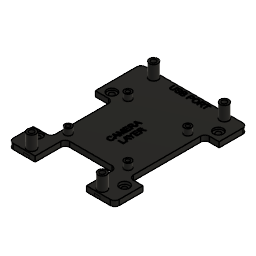
BATTERY-CAMERA_SPACER (Autodesk Fusion 360 design; units mm, degrees)
part number: 2026-05-13-14-17-40-466
Autodesk Fusion 360 part; units mm, degrees
note: some values were not read from the file. Chosen so that the rebuilt part matches the saved one: that a step has no effect; the layout of a text.
sketch "Sketch1" plane through (0, 0, 0) normal (0, 0, 1) x (1, 0, 0)
  line L0 (2.5, 0) -> (57.5, 0)
  line L1 (60, 2.5) -> (60, 72.5)
  line L2 (57.5, 75) -> (2.5, 75)
  line L3 (0, 72.5) -> (0, 2.5)
  arc A0 (2.5, 75) -> (0, 72.5) centre (2.5, 72.5) ccw
  arc A1 (60, 72.5) -> (57.5, 75) centre (57.5, 72.5) ccw
  arc A2 (57.5, 0) -> (60, 2.5) centre (57.5, 2.5) ccw
  arc A3 (0, 2.5) -> (2.5, 0) centre (2.5, 2.5) ccw
  point P0 (60, 0)
  point P1 (0, 75)
  dimension "d1" = 60
  dimension "d2" = 75
  dimension "d3" = 2.5
  constraint horizontal L0
  constraint vertical L1
  constraint horizontal L2
  constraint vertical L3
  constraint coincident P1 L2
  constraint coincident P1 L3
  constraint tangent L2 A0
  constraint tangent L3 A0
  constraint tangent L1 A1
  constraint tangent L2 A1
  constraint equal A0 A1
  constraint coincident P0 L0
  constraint coincident P0 L1
  constraint tangent L0 A2
  constraint tangent L1 A2
  constraint equal A0 A2
  constraint coincident origin L0
  constraint coincident origin L3
  constraint tangent L0 A3
  constraint tangent L3 A3
  constraint equal A0 A3
  measures "d1" distance of origin P0
  measures "d2" distance of origin P1
  measures "d3" radius of A0
extrude "Extrude1" add sketch "Sketch1" along normal blind 3
sketch "Sketch2" plane through (0, 0, 3) normal (0, 0, 1) x (-1, 0, 0)
  arc A0 (0, -2.5) -> (-2.5, 0) centre (-2.5, -2.5) ccw
  line L0 (-2.5, 0) -> (-57.5, 0)
  arc A1 (-57.5, 0) -> (-60, -2.5) centre (-57.5, -2.5) ccw
  line L1 (-60, -2.5) -> (-60, -72.5)
  arc A2 (-60, -72.5) -> (-57.5, -75) centre (-57.5, -72.5) ccw
  line L2 (-57.5, -75) -> (-2.5, -75)
  arc A3 (-2.5, -75) -> (0, -72.5) centre (-2.5, -72.5) ccw
  line L3 (0, -72.5) -> (0, -2.5)
  circle A4 centre (-50, -72) radius 1.4
  circle A5 centre (-50, -72) radius 2.5
  circle A6 centre (-10, -72) radius 1.4
  circle A7 centre (-10, -72) radius 2.5
  circle A8 centre (-50, -3) radius 1.4
  circle A9 centre (-50, -3) radius 2.5
  circle A10 centre (-10, -3) radius 1.4
  circle A11 centre (-10, -3) radius 2.5
  dimension "d6" = 2.8
  dimension "d7" = 5
  dimension "d8" = 10
  dimension "d9" = 3
  dimension "d10" = 2.8
  dimension "d11" = 5
  dimension "d12" = 3
  dimension "d13" = 10
  dimension "d14" = 2.8
  dimension "d15" = 5
  dimension "d16" = 3
  dimension "d17" = 10
  dimension "d18" = 2.8
  dimension "d19" = 5
  dimension "d20" = 10
  dimension "d21" = 3
  constraint concentric A4 A5
  constraint concentric A6 A7
  constraint concentric A8 A9
  constraint concentric A10 A11
  measures "d6" diameter of A4
  measures "d7" diameter of A5
  measures "d8" distance of L1 A4.centre
  measures "d9" distance of L2 A4.centre
  measures "d10" diameter of A6
  measures "d11" diameter of A7
  measures "d12" distance of L2 A6.centre
  measures "d13" distance of L3 A6.centre
  measures "d14" diameter of A8
  measures "d15" diameter of A9
  measures "d16" distance of L0 A8.centre
  measures "d17" distance of L1 A8.centre
  measures "d18" diameter of A10
  measures "d19" diameter of A11
  measures "d20" distance of L3 A10.centre
  measures "d21" distance of L0 A10.centre
extrude "Extrude2" cut sketch "Sketch2" against normal blind 6 contours A4 | A6 | A8 | A10
extrude "Extrude3" add sketch "Sketch2" along normal blind 8 contours A5 | A7 | A9 | A11
sketch "Sketch3" plane through (0, 0, 3) normal (0, 0, 1) x (-1, 0, 0)
  line L0 (-17, -70) -> (-44, -70) construction
  line L1 (-44, -70) -> (-44, -75) construction
  line L2 (-44, -75) -> (-17, -75) construction
  line L3 (-17, -75) -> (-17, -70) construction
  line L4 (-36.7995, -28.0303) -> (-36.8426, -50.0364) construction
  line L5 (-36.8426, -50.0364) -> (-24.5082, -50.0606) construction
  line L6 (-24.5082, -50.0606) -> (-24.4651, -28.0545) construction
  line L7 (-24.4651, -28.0545) -> (-36.7995, -28.0303) construction
  dimension "d26" = 3
  dimension "d28" = 3
  text T0 "USB PORT" font "Arial" height 3 align centre middle in box 27 x 5 at (-17, -70) x (-1, 0) y (0, -1) spacing 1
extrude "Extrude4" [no effect]
sketch "Sketch13" plane through (0, 0, 3) normal (0, 0, 1) x (-1, 0, 0)
  circle A0 centre (-5.4, -11) radius 1.4
  circle A1 centre (-5.4, -11) radius 2.75
  line L0 (0, -72.5) -> (0, -2.5)
  line L1 (-2.5, 0) -> (-57.5, 0)
  circle A2 centre (-54.6, -11) radius 1.4
  circle A3 centre (-54.6, -11) radius 2.75
  line L2 (-60, -2.5) -> (-60, -72.5)
  circle A4 centre (-5.4, -53) radius 1.4
  circle A5 centre (-5.4, -53) radius 2.75
  line L3 (-57.5, -75) -> (-2.5, -75)
  circle A6 centre (-54.6, -64) radius 1.4
  circle A7 centre (-54.6, -64) radius 2.75
  dimension "d67" = 2.8
  dimension "d68" = 5.5
  dimension "d69" = 5.4
  dimension "d70" = 11
  dimension "d71" = 2.8
  dimension "d72" = 5.5
  dimension "d73" = 11
  dimension "d74" = 5.4
  dimension "d75" = 2.8
  dimension "d76" = 5.5
  dimension "d77" = 5.4
  dimension "d78" = 22
  dimension "d79" = 2.8
  dimension "d80" = 5.5
  dimension "d81" = 5.4
  dimension "d82" = 11
  constraint concentric A0 A1
  constraint concentric A2 A3
  constraint concentric A4 A5
  constraint concentric A6 A7
  measures "d67" diameter of A0
  measures "d68" diameter of A1
  measures "d69" distance of A0.centre L0
  measures "d70" distance of A0.centre L1
  measures "d71" diameter of A2
  measures "d72" diameter of A3
  measures "d73" distance of L1 A2.centre
  measures "d74" distance of A2.centre L2
  measures "d75" diameter of A4
  measures "d76" diameter of A5
  measures "d77" distance of L0 A4.centre
  measures "d78" distance of A4.centre L3
  measures "d79" diameter of A6
  measures "d80" diameter of A7
  measures "d81" distance of L2 A6.centre
  measures "d82" distance of L3 A6.centre
extrude "Extrude11" cut sketch "Sketch13" against normal blind 3 contours A0 | A2 | A4 | A6
extrude "Extrude12" cut sketch "Sketch13" against normal blind 1.5 contours A3
sketch "Sketch14" plane through (0, 0, 0) normal (0, 0, -1) x (1, 0, 0)
  arc A0 (2.5, 0) -> (0, -2.5) centre (2.5, -2.5) ccw
  line L0 (0, -2.5) -> (0, -72.5)
  arc A1 (0, -72.5) -> (2.5, -75) centre (2.5, -72.5) ccw
  line L1 (2.5, -75) -> (57.5, -75)
  arc A2 (57.5, -75) -> (60, -72.5) centre (57.5, -72.5) ccw
  line L2 (60, -72.5) -> (60, -2.5)
  arc A3 (60, -2.5) -> (57.5, 0) centre (57.5, -2.5) ccw
  line L3 (57.5, 0) -> (2.5, 0)
  circle A4 centre (10, -3) radius 1.4
  circle A5 centre (10, -72) radius 1.4
  circle A6 centre (50, -3) radius 1.4
  circle A7 centre (50, -72) radius 1.4
  circle A8 centre (54.6, -64) radius 1.4
  circle A9 centre (54.6, -11) radius 1.4
  circle A10 centre (5.4, -53) radius 1.4
  circle A11 centre (5.4, -11) radius 1.4
  line L4 (50.8083, -4.4) -> (51.6166, -3)
  line L5 (51.6166, -3) -> (50.8083, -1.6)
  line L6 (50.8083, -1.6) -> (49.1917, -1.6)
  line L7 (49.1917, -1.6) -> (48.3834, -3)
  line L8 (48.3834, -3) -> (49.1917, -4.4)
  line L9 (49.1917, -4.4) -> (50.8083, -4.4)
  line L10 (51.5305, -5.7162) -> (53.1175, -3.0327)
  line L11 (53.1175, -3.0327) -> (51.587, -0.3165)
  line L12 (51.587, -0.3165) -> (48.4695, -0.2838)
  line L13 (48.4695, -0.2838) -> (46.8825, -2.9673)
  line L14 (46.8825, -2.9673) -> (48.413, -5.6835)
  line L15 (48.413, -5.6835) -> (51.5305, -5.7162)
  line L16 (10.7939, -4.4082) -> (11.6165, -3.0166)
  line L17 (11.6165, -3.0166) -> (10.8226, -1.6084)
  line L18 (10.8226, -1.6084) -> (9.2061, -1.5918)
  line L19 (9.2061, -1.5918) -> (8.3835, -2.9834)
  line L20 (8.3835, -2.9834) -> (9.1774, -4.3916)
  line L21 (9.1774, -4.3916) -> (10.7939, -4.4082)
  line L22 (11.5588, -5.7) -> (13.1177, -3)
  line L23 (13.1177, -3) -> (11.5588, -0.3)
  line L24 (11.5588, -0.3) -> (8.4412, -0.3)
  line L25 (8.4412, -0.3) -> (6.8823, -3)
  line L26 (6.8823, -3) -> (8.4412, -5.7)
  line L27 (8.4412, -5.7) -> (11.5588, -5.7)
  line L28 (9.1917, -70.6) -> (8.3834, -72)
  line L29 (8.3834, -72) -> (9.1917, -73.4)
  line L30 (9.1917, -73.4) -> (10.8083, -73.4)
  line L31 (10.8083, -73.4) -> (11.6166, -72)
  line L32 (11.6166, -72) -> (10.8083, -70.6)
  line L33 (10.8083, -70.6) -> (9.1917, -70.6)
  line L34 (8.4412, -69.3) -> (6.8823, -72)
  line L35 (6.8823, -72) -> (8.4412, -74.7)
  line L36 (8.4412, -74.7) -> (11.5588, -74.7)
  line L37 (11.5588, -74.7) -> (13.1177, -72)
  line L38 (13.1177, -72) -> (11.5588, -69.3)
  line L39 (11.5588, -69.3) -> (8.4412, -69.3)
  line L40 (49.1917, -70.6) -> (48.3834, -72)
  line L41 (48.3834, -72) -> (49.1917, -73.4)
  line L42 (49.1917, -73.4) -> (50.8083, -73.4)
  line L43 (50.8083, -73.4) -> (51.6166, -72)
  line L44 (51.6166, -72) -> (50.8083, -70.6)
  line L45 (50.8083, -70.6) -> (49.1917, -70.6)
  line L46 (48.4412, -69.3) -> (46.8823, -72)
  line L47 (46.8823, -72) -> (48.4412, -74.7)
  line L48 (48.4412, -74.7) -> (51.5588, -74.7)
  line L49 (51.5588, -74.7) -> (53.1177, -72)
  line L50 (53.1177, -72) -> (51.5588, -69.3)
  line L51 (51.5588, -69.3) -> (48.4412, -69.3)
  point P0 (50, -3)
  point P1 (50, -3)
  point P2 (10, -3)
  point P3 (10, -3)
  point P4 (10, -72)
  point P5 (10, -72)
  point P6 (50, -72)
  point P7 (50, -72)
  dimension "d87" = 1.4
  dimension "d88" = 2.7
  dimension "d89" = 1.4
  dimension "d90" = 2.7
  dimension "d91" = 1.4
  dimension "d92" = 2.7
  dimension "d93" = 1.4
  dimension "d94" = 2.7
  constraint coincident P1 P0
  constraint coincident P3 P2
  constraint coincident P5 P4
  constraint coincident P7 P6
  measures "d87" distance of P1 L9
  measures "d88" distance of P1 L15
  measures "d89" distance of P3 L21
  measures "d90" distance of P3 L27
  measures "d91" distance of P5 L33
  measures "d92" distance of P5 L39
  measures "d93" distance of P7 L45
  measures "d94" distance of P7 L51
extrude "Extrude13" cut sketch "Sketch14" against normal blind 1.5 contours A4 L16 L17 | A4 L17 L18 | A4 L16 L21 | A4 L18 L19 | A4 L20 L21 | A4 L19 L20 | A5 L31 L32 | A5 L32 L33 | A5 L30 L31 | A5 L28 L33 | A5 L29 L30 | A5 L28 L29 | A6 L4 L5 | A6 L5 L6 | A6 L4 L9 | A6 L6 L7 | A6 L8 L9 | A6 L7 L8 | A7 L43 L44 | A7 L44 L45 | A7 L42 L43 | A7 L40 L45 | A7 L41 L42 | A7 L40 L41 | L10 L11 L12 L13 L14 L15 | L22 L23 L24 L25 L26 L27 | L34 L35 L36 L37 L38 L39 | L46 L47 L48 L49 L50 L51
sketch "Sketch15" plane through (0, 0, 3) normal (0, 0, 1) x (-1, 0, 0)
  line L0 (-11, -18.5) -> (-49, -18.5)
  line L1 (-49, -18.5) -> (-49, -56.5)
  line L2 (-49, -56.5) -> (-11, -56.5)
  line L3 (-11, -56.5) -> (-11, -18.5)
  line L4 (-2.5, 0) -> (-57.5, 0)
  line L5 (0, -72.5) -> (0, -2.5)
  circle A0 centre (-13.1, -20.6) radius 1.1
  circle A1 centre (-46.9, -20.6) radius 1.1
  circle A2 centre (-46.9, -54.4) radius 1.1
  circle A3 centre (-13.1, -54.4) radius 1.1
  circle A4 centre (-13.1, -20.6) radius 2
  circle A5 centre (-13.1, -54.4) radius 2
  circle A6 centre (-46.9, -54.4) radius 2
  circle A7 centre (-46.9, -20.6) radius 2
  dimension "d97" = 38
  dimension "d98" = 38
  dimension "d99" = 18.5
  dimension "d100" = 11
  dimension "d101" = 2.2
  dimension "d102" = 2.1
  dimension "d103" = 2.1
  dimension "d104" = 2.2
  dimension "d105" = 2.1
  dimension "d106" = 2.1
  dimension "d107" = 2.2
  dimension "d108" = 2.1
  dimension "d109" = 2.1
  dimension "d110" = 2.2
  dimension "d111" = 2.1
  dimension "d112" = 2.1
  dimension "d123" = 4
  dimension "d124" = 4
  dimension "d125" = 4
  dimension "d126" = 4
  constraint horizontal L0
  constraint vertical L1
  constraint horizontal L2
  constraint vertical L3
  constraint concentric A0 A4
  constraint concentric A3 A5
  constraint concentric A2 A6
  constraint concentric A1 A7
  measures "d97" distance of L0.start L0.end
  measures "d98" distance of L0.start L2.end
  measures "d99" distance of L0 L4
  measures "d100" distance of L3 L5
  measures "d101" diameter of A0
  measures "d102" distance of L3 A0.centre
  measures "d103" distance of L0 A0.centre
  measures "d104" diameter of A1
  measures "d105" distance of L0 A1.centre
  measures "d106" distance of L1 A1.centre
  measures "d107" diameter of A2
  measures "d108" distance of L1 A2.centre
  measures "d109" distance of L2 A2.centre
  measures "d110" diameter of A3
  measures "d111" distance of L2 A3.centre
  measures "d112" distance of L3 A3.centre
  measures "d123" diameter of A4
  measures "d124" diameter of A5
  measures "d125" diameter of A6
  measures "d126" diameter of A7
extrude "Extrude14" cut sketch "Sketch15" against normal blind 3 contours A0 | A1 | A2 | A3
sketch "Sketch16" plane through (0, 0, 3) normal (0, 0, 1) x (-1, 0, 0)
  line L0 (0, -14) -> (-7.5, -14)
  line L1 (-10, -16.5) -> (-10, -46.5)
  line L2 (-7.5, -49) -> (0, -49)
  line L3 (0, -49) -> (0, -14)
  arc A0 (-7.5, -14) -> (-10, -16.5) centre (-7.5, -16.5) ccw
  arc A1 (-10, -46.5) -> (-7.5, -49) centre (-7.5, -46.5) ccw
  line L4 (-15, 0) -> (-44, 0)
  line L5 (-44, 0) -> (-44, -14.5)
  line L6 (-41.5, -17) -> (-17.5, -17)
  line L7 (-15, -14.5) -> (-15, 0)
  arc A2 (-17.5, -17) -> (-15, -14.5) centre (-17.5, -14.5) ccw
  arc A3 (-44, -14.5) -> (-41.5, -17) centre (-41.5, -14.5) ccw
  line L8 (-60, -16) -> (-54.5, -16)
  line L9 (-52, -18.5) -> (-52, -56.5)
  line L10 (-54.5, -59) -> (-60, -59)
  line L11 (-60, -59) -> (-60, -16)
  arc A4 (-52, -18.5) -> (-54.5, -16) centre (-54.5, -18.5) ccw
  arc A5 (-54.5, -59) -> (-52, -56.5) centre (-54.5, -56.5) ccw
  point P0 (-10, -14)
  point P1 (-5.4, -11)
  point P2 (-52, -16)
  dimension "d115" = 10
  dimension "d116" = 35
  dimension "d117" = 3
  dimension "d118" = 2.5
  dimension "d120" = 2.5
  dimension "d131" = 8
  dimension "d132" = 2.5
  constraint horizontal L0
  constraint vertical L1
  constraint horizontal L2
  constraint vertical L3
  constraint coincident P0 L0
  constraint coincident P0 L1
  constraint tangent L0 A0
  constraint tangent L1 A0
  constraint tangent L1 A1
  constraint tangent L2 A1
  constraint equal A0 A1
  constraint horizontal L4
  constraint vertical L5
  constraint horizontal L6
  constraint vertical L7
  constraint tangent L6 A2
  constraint tangent L7 A2
  constraint tangent L5 A3
  constraint tangent L6 A3
  constraint equal A2 A3
  constraint horizontal L8
  constraint vertical L9
  constraint horizontal L10
  constraint vertical L11
  constraint coincident P2 L8
  constraint coincident P2 L9
  constraint tangent L8 A4
  constraint tangent L9 A4
  constraint tangent L9 A5
  constraint tangent L10 A5
  constraint equal A4 A5
  measures "d115" distance of L0.start P0
  measures "d116" distance of L0.start L2.end
  measures "d117" distance of L0 P1
  measures "d118" radius of A0
  measures "d120" radius of A2
  measures "d131" distance of L8.start P2
  measures "d132" radius of A4
extrude "Extrude16" add sketch "Sketch15" along normal blind 3.5 contours A4 | A5 | A6 | A7
extrude "Extrude17" cut sketch "Sketch13" against normal blind 1 contours A1 | A5 | A7
extrude "Extrude18" cut sketch "Sketch16" against normal blind 3
sketch "Sketch19" plane through (0, 0, 3) normal (0, 0, 1) x (-1, 0, 0)
  line L0 (-54.5, -59) -> (-60, -59)
  line L1 (-60, -59) -> (-60, -72.5)
  arc A0 (-60, -72.5) -> (-57.5, -75) centre (-57.5, -72.5) ccw
  line L2 (-57.5, -75) -> (-2.5, -75)
  arc A1 (-2.5, -75) -> (0, -72.5) centre (-2.5, -72.5) ccw
  line L3 (0, -72.5) -> (0, -49)
  line L4 (0, -49) -> (-7.5, -49)
  arc A2 (-10, -46.5) -> (-7.5, -49) centre (-7.5, -46.5) ccw
  line L5 (-10, -46.5) -> (-10, -16.5)
  arc A3 (-7.5, -14) -> (-10, -16.5) centre (-7.5, -16.5) ccw
  line L6 (-7.5, -14) -> (0, -14)
  line L7 (0, -14) -> (0, -2.5)
  arc A4 (0, -2.5) -> (-2.5, 0) centre (-2.5, -2.5) ccw
  line L8 (-2.5, 0) -> (-15, 0)
  line L9 (-15, 0) -> (-15, -14.5)
  arc A5 (-17.5, -17) -> (-15, -14.5) centre (-17.5, -14.5) ccw
  line L10 (-17.5, -17) -> (-41.5, -17)
  arc A6 (-44, -14.5) -> (-41.5, -17) centre (-41.5, -14.5) ccw
  line L11 (-44, -14.5) -> (-44, 0)
  line L12 (-44, 0) -> (-57.5, 0)
  arc A7 (-57.5, 0) -> (-60, -2.5) centre (-57.5, -2.5) ccw
  line L13 (-60, -2.5) -> (-60, -16)
  line L14 (-60, -16) -> (-54.5, -16)
  arc A8 (-52, -18.5) -> (-54.5, -16) centre (-54.5, -18.5) ccw
  line L15 (-52, -18.5) -> (-52, -56.5)
  arc A9 (-54.5, -59) -> (-52, -56.5) centre (-54.5, -56.5) ccw
  circle A10 centre (-54.6, -64) radius 2.75
  circle A11 centre (-5.4, -53) radius 2.75
  circle A12 centre (-5.4, -11) radius 2.75
  circle A13 centre (-13.1, -54.4) radius 2
  circle A14 centre (-13.1, -20.6) radius 2
  circle A15 centre (-54.6, -11) radius 2.75
  circle A16 centre (-10, -3) radius 2.5
  circle A17 centre (-10, -72) radius 2.5
  circle A18 centre (-50, -3) radius 2.5
  circle A19 centre (-50, -72) radius 2.5
  circle A20 centre (-46.9, -54.4) radius 2
  circle A21 centre (-46.9, -20.6) radius 2
  line L16 (-40, -25) -> (-40, -50) construction
  line L17 (-40, -50) -> (-20, -50) construction
  line L18 (-20, -50) -> (-20, -25) construction
  line L19 (-20, -25) -> (-40, -25) construction
  line L20 (-15, -70) -> (-45, -70) construction
  line L21 (-45, -70) -> (-45, -75) construction
  line L22 (-45, -75) -> (-15, -75) construction
  line L23 (-15, -75) -> (-15, -70) construction
  dimension "d135" = 3
  dimension "d137" = 3
  text T0 "CAMERA\nLAYER" font "Arial" height 3 align centre middle in box 25 x 20 at (-40, -25) x (0, -1) y (1, 0) spacing 1 kerned
  text T1 "USB PORT" font "Arial" height 3 align centre middle in box 30 x 5 at (-15, -70) x (-1, 0) y (0, -1) spacing 1 kerned
extrude "Extrude19" cut sketch "Sketch19" against normal blind 2 text T0 T1
sketch "Sketch20" plane through (0, 0, 0) normal (0, 0, -1) x (1, 0, 0)
  line L0 (60, -59) -> (54.5, -59)
  arc A0 (52, -56.5) -> (54.5, -59) centre (54.5, -56.5) ccw
  line L1 (52, -56.5) -> (52, -18.5)
  arc A1 (54.5, -16) -> (52, -18.5) centre (54.5, -18.5) ccw
  line L2 (54.5, -16) -> (60, -16)
  line L3 (60, -16) -> (60, -2.5)
  arc A2 (60, -2.5) -> (57.5, 0) centre (57.5, -2.5) ccw
  line L4 (57.5, 0) -> (44, 0)
  line L5 (44, 0) -> (44, -14.5)
  arc A3 (41.5, -17) -> (44, -14.5) centre (41.5, -14.5) ccw
  line L6 (41.5, -17) -> (17.5, -17)
  arc A4 (15, -14.5) -> (17.5, -17) centre (17.5, -14.5) ccw
  line L7 (15, -14.5) -> (15, 0)
  line L8 (15, 0) -> (2.5, 0)
  arc A5 (2.5, 0) -> (0, -2.5) centre (2.5, -2.5) ccw
  line L9 (0, -2.5) -> (0, -14)
  line L10 (0, -14) -> (7.5, -14)
  arc A6 (10, -16.5) -> (7.5, -14) centre (7.5, -16.5) ccw
  line L11 (10, -16.5) -> (10, -46.5)
  arc A7 (7.5, -49) -> (10, -46.5) centre (7.5, -46.5) ccw
  line L12 (7.5, -49) -> (0, -49)
  line L13 (0, -49) -> (0, -72.5)
  arc A8 (0, -72.5) -> (2.5, -75) centre (2.5, -72.5) ccw
  line L14 (2.5, -75) -> (57.5, -75)
  arc A9 (57.5, -75) -> (60, -72.5) centre (57.5, -72.5) ccw
  line L15 (60, -72.5) -> (60, -59)
  circle A10 centre (46.9, -20.6) radius 1.1
  circle A11 centre (13.1, -20.6) radius 1.1
  circle A12 centre (46.9, -54.4) radius 1.1
  circle A13 centre (13.1, -54.4) radius 1.1
  circle A14 centre (5.4, -11) radius 1.4
  circle A15 centre (5.4, -53) radius 1.4
  circle A16 centre (54.6, -11) radius 1.4
  circle A17 centre (54.6, -64) radius 1.4
  line L16 (46.8823, -72) -> (48.4412, -69.3)
  line L17 (48.4412, -69.3) -> (51.5588, -69.3)
  line L18 (51.5588, -69.3) -> (53.1177, -72)
  line L19 (53.1177, -72) -> (51.5588, -74.7)
  line L20 (51.5588, -74.7) -> (48.4412, -74.7)
  line L21 (48.4412, -74.7) -> (46.8823, -72)
  line L22 (53.1175, -3.0327) -> (51.5305, -5.7162)
  line L23 (51.5305, -5.7162) -> (48.413, -5.6835)
  line L24 (48.413, -5.6835) -> (46.8825, -2.9673)
  line L25 (46.8825, -2.9673) -> (48.4695, -0.2838)
  line L26 (48.4695, -0.2838) -> (51.587, -0.3165)
  line L27 (51.587, -0.3165) -> (53.1175, -3.0327)
  line L28 (6.8823, -72) -> (8.4412, -69.3)
  line L29 (8.4412, -69.3) -> (11.5588, -69.3)
  line L30 (11.5588, -69.3) -> (13.1177, -72)
  line L31 (13.1177, -72) -> (11.5588, -74.7)
  line L32 (11.5588, -74.7) -> (8.4412, -74.7)
  line L33 (8.4412, -74.7) -> (6.8823, -72)
  line L34 (13.1177, -3) -> (11.5588, -5.7)
  line L35 (11.5588, -5.7) -> (8.4412, -5.7)
  line L36 (8.4412, -5.7) -> (6.8823, -3)
  line L37 (6.8823, -3) -> (8.4412, -0.3)
  line L38 (8.4412, -0.3) -> (11.5588, -0.3)
  line L39 (11.5588, -0.3) -> (13.1177, -3)
  line L40 (46.1784, -23.7516) -> (49.2686, -22.8007)
  line L41 (49.2686, -22.8007) -> (49.9902, -19.6491)
  line L42 (49.9902, -19.6491) -> (47.6216, -17.4484)
  line L43 (47.6216, -17.4484) -> (44.5314, -18.3993)
  line L44 (44.5314, -18.3993) -> (43.8098, -21.5509)
  line L45 (43.8098, -21.5509) -> (46.1784, -23.7516)
  line L46 (43.8431, -53.347) -> (44.4596, -56.5208)
  line L47 (44.4596, -56.5208) -> (47.5165, -57.5738)
  line L48 (47.5165, -57.5738) -> (49.9569, -55.453)
  line L49 (49.9569, -55.453) -> (49.3404, -52.2792)
  line L50 (49.3404, -52.2792) -> (46.2835, -51.2262)
  line L51 (46.2835, -51.2262) -> (43.8431, -53.347)
  line L52 (10.099, -53.1971) -> (10.5577, -56.3975)
  line L53 (10.5577, -56.3975) -> (13.5588, -57.6004)
  line L54 (13.5588, -57.6004) -> (16.101, -55.6029)
  line L55 (16.101, -55.6029) -> (15.6423, -52.4025)
  line L56 (15.6423, -52.4025) -> (12.6412, -51.1996)
  line L57 (12.6412, -51.1996) -> (10.099, -53.1971)
  line L58 (10.3, -22.2166) -> (13.1, -23.8332)
  line L59 (13.1, -23.8332) -> (15.9, -22.2166)
  line L60 (15.9, -22.2166) -> (15.9, -18.9834)
  line L61 (15.9, -18.9834) -> (13.1, -17.3668)
  line L62 (13.1, -17.3668) -> (10.3, -18.9834)
  line L63 (10.3, -18.9834) -> (10.3, -22.2166)
  point P0 (46.9, -20.6)
  point P1 (46.9, -54.4)
  point P2 (13.1, -54.4)
  point P3 (13.1, -20.6)
  dimension "d141" = 2.8
  dimension "d142" = 2.8
  dimension "d143" = 2.8
  dimension "d144" = 2.8
  constraint coincident P0 A10.centre
  constraint coincident P1 A12.centre
  constraint coincident P2 A13.centre
  constraint coincident P3 A11.centre
  measures "d141" distance of P0 L45
  measures "d142" distance of P1 L51
  measures "d143" distance of P2 L57
  measures "d144" distance of P3 L63
extrude "Extrude20" cut sketch "Sketch20" against normal blind 1.5 contours L40 L41 L42 L43 L44 L45 | L46 L47 L48 L49 L50 L51 | L52 L53 L54 L55 L56 L57 | L58 L59 L60 L61 L62 L63
equation "d27 = 'USB PORT'"
equation "d29 = 'CAMERA LAYER'"
equation "d136 = 'CAMERA LAYER'"
equation "d138 = 'USB PORT'"
